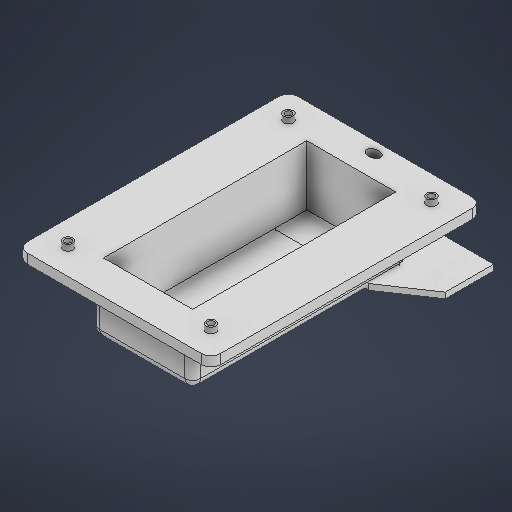
# Autodesk Inventor part: body
Saved by Autodesk Inventor 2027 (Build 310192000, 192)
## iProperties
Created: 2026-05-11
Part Number: body
Material: Generic
Document SubType Name: Modeling
Designer: maksi
Density: 1 g/cm^3
Appearance: Default
Author: maksi
Autodesk Inventor part; units mm, degrees
ref_plane "YZ Plane" through (0, 0, 0) normal (1, 0, 0) x (0, 1, 0)
ref_plane "XZ Plane" through (0, 0, 0) normal (0, 1, 0) x (-1, 0, 0)
ref_plane "XY Plane" through (0, 0, 0) normal (0, 0, 1) x (1, 0, 0)
sketch "Sketch1" plane through (0, 0, 0) normal (0, 1, 0) x (-1, 0, 0)
  line L0 (-40, 60) -> (40, 60)
  line L1 (40, 60) -> (40, -60)
  line L2 (40, -60) -> (-40, -60)
  line L3 (-40, -60) -> (-40, 60)
  line L4 (-40, 60) -> (40, -60) construction
  line L5 (40, 60) -> (-40, -60) construction
  line L6 (40, -60) -> (38.6, -60) construction
  line L7 (38.6, -60) -> (38.6, -58.6) construction
  line L8 (38.6, -58.6) -> (40, -58.6) construction
  line L9 (40, -58.6) -> (40, -60) construction
  line L10 (38.6, -58.6) -> (35.3, -58.6) construction
  line L11 (35.3, -58.6) -> (35.3, -55.3) construction
  line L12 (35.3, -55.3) -> (38.6, -55.3) construction
  line L13 (38.6, -55.3) -> (38.6, -58.6) construction
  circle A0 centre (36.95, -56.95) radius 1.65
  circle A1 centre (-36.95, -56.95) radius 1.65
  circle A2 centre (36.95, 56.95) radius 1.65
  circle A3 centre (-36.95, 56.95) radius 1.65
  line L14 (50, -70) -> (50, 70)
  line L15 (50, 70) -> (-50, 70)
  line L16 (-50, 70) -> (-50, -70)
  line L17 (-50, -70) -> (50, -70)
  line L18 (-23, 52.5) -> (23, 52.5)
  line L19 (23, 52.5) -> (23, -52.5)
  line L20 (23, -52.5) -> (-23, -52.5)
  line L21 (-23, -52.5) -> (-23, 52.5)
  line L22 (-23, 52.5) -> (23, -52.5) construction
  line L23 (23, 52.5) -> (-23, -52.5) construction
  point P0 (0, 0)
  dimension "d0" = 80
  dimension "d1" = 120
  dimension "d2" = 1.4
  dimension "d3" = 1.4
  dimension "d4" = 3.3
  dimension "d5" = 3.3
  dimension "d6" = 3.3
  dimension "d9" = 73.9
  dimension "d12" = 113.9
  dimension "d15" = 10
  dimension "d16" = 46
  dimension "d17" = 105
  constraints: 48 end point, 10 parallel, 5 horizontal, 5 perpendicular, 4 centre point, 4 midpoint, 2 tangent, 1 vertical, 9 other
  measures "d0" distance of L1.end L2.end
  measures "d1" distance of L0.end L1.end
  measures "d2" distance of L7.end L8.end
  measures "d3" distance of L6.end L7.end
  measures "d4" distance of L11.end L12.end
  measures "d5" distance of L10.end L11.end
  measures "d6" diameter of A0
  measures "d9" distance of A0.centre A1.centre
  measures "d12" distance of A0.centre A2.centre
  measures "d15" distance between parallel lines of L1 L14
  measures "d16" distance of L19.end L20.end
  measures "d17" distance of L18.end L19.end
extrude "Extrusion1" add sketch "Sketch1" along normal blind 5 contours L0 L1 L2 L3 | L17 L16 L15 L14
sketch "Sketch2" plane through (-50, 0, 70) normal (0, 0, 1) x (1, 0, 0)
  line L0 (73, 0) -> (27, 0) projected
  line L1 (27, 0) -> (73, 0)
  line L2 (73, 0) -> (73, -26)
  line L3 (73, -26) -> (27, -26)
  line L4 (27, -26) -> (27, 0)
  line L5 (0, 0) -> (100, 0) projected
  line L6 (24, 3) -> (76, 3)
  line L7 (76, 3) -> (76, -25)
  line L8 (72, -29) -> (28, -29)
  line L9 (24, -25) -> (24, 3)
  arc A0 (24, -25) -> (28, -29) centre (28, -25) ccw
  arc A1 (72, -29) -> (76, -25) centre (72, -25) ccw
  point P0 (50, 0)
  point P1 (24, 0)
  point P2 (76, 0)
  dimension "d20" = 26
  dimension "d21" = 3
  dimension "d22" = 4
  constraints: 16 end point, 4 parallel, 4 point on circle, 4 tangent, 2 centre point, 2 perpendicular, 1 collinear, 1 equal radius, 3 other
  measures "d20" distance of L0.start L2.end
  measures "d21" distance between parallel lines of L4 L9
  measures "d22" radius of A0
extrude "Extrusion2" add sketch "Sketch2" against normal up to surface (105 mm away) from surface at -17.5 contours L5 L7 A1 L8 A0 L9 L4 L3 L2
sketch "Sketch3" plane through (23, -26, -52.5) normal (0, 0, -1) x (-1, 0, 0)
  line L0 (-3, 26) -> (-3, 1) projected
  arc A0 (-3, 1) -> (1, -3) centre (1, 1) ccw projected
  line L1 (1, -3) -> (45, -3) projected
  arc A1 (45, -3) -> (49, 1) centre (45, 1) ccw projected
  line L2 (49, 1) -> (49, 26) projected
  line L3 (46, 26) -> (0, 26) projected
  line L4 (-3, 26) -> (0, 26) projected
  line L5 (46, 26) -> (49, 26) projected
  point P0 (23, 26)
extrude "Extrusion3" add sketch "Sketch3" along normal blind 3
extrude "Extrusion4" add sketch "Sketch3" against normal blind 3 from surface at -105
fillet "Fillet1" radius 4 10 edges at (26, -12.5, 55.5) (0, -29, 55.5) (-24.8284, -27.8284, 55.5) (-26, -12.5, 55.5) (24.8284, -27.8284, 55.5) (0, -29, -55.5) (-24.8284, -27.8284, -55.5) (-26, -12.5, -55.5) (26, -12.5, -55.5) (24.8284, -27.8284, -55.5)
sketch "Sketch4" plane through (0, 5, 0) normal (0, 1, 0) x (1, 0, 0)
  circle A0 centre (-36.95, 56.95) radius 1.65 projected
  circle A1 centre (-36.95, 56.95) radius 2.5
  circle A2 centre (-36.95, 56.95) radius 1.65
  point P0 (0, 0)
  dimension "d30" = 5
  constraints: 2 centre point, 2 coincident
  measures "d30" diameter of A1
extrude "Extrusion5" add sketch "Sketch4" along normal blind 3
pattern_linear "Rectangular Pattern1" count 2 spacing 73.9 along (1, 0, 0) count 2 spacing 113.9 along (0, 0, 1) of "Extrusion5"
fillet "Fillet2" radius 5 4 edges at (-50, 2.5, 70) (-50, 2.5, -70) (50, 2.5, -70) (50, 2.5, 70)
sketch "Sketch5" plane through (-22, -29, -51.5) normal (0, -1, 0) x (1, 0, 0)
  line L0 (44, 0) -> (44, -4) projected
  line L1 (44, 0) -> (71.6, 0)
  line L2 (71.6, 0) -> (71.6, -25)
  line L3 (71.6, -25) -> (44, -25)
  line L4 (44, -25) -> (44, 0)
  line L5 (44, 0) -> (0, 0) projected
  line L6 (0, 0) -> (-27.6, 0)
  line L7 (-27.6, 0) -> (-27.6, -25)
  line L8 (-27.6, -25) -> (0, -25)
  line L9 (0, -25) -> (0, 0)
  line L10 (44, -25) -> (0, -25)
  line L11 (0, -25) -> (0, 0)
  line L12 (0, 0) -> (44, 0)
  line L13 (44, 0) -> (44, -25)
  line L14 (44, -25) -> (0, 0) construction
  line L15 (0, -25) -> (44, 0) construction
  ellipse E0 centre (22, -12.5) end of major axis (18.3001, -12.5) minor radius 2.5167
  line L16 (-1, -1) -> (45, -1) projected
  line L17 (0, 0) -> (-4, 0) projected
  line L18 (0, 103) -> (0, 0) projected
  line L19 (-4, 103) -> (0, 103) projected
  line L20 (-4, 103) -> (-4, 0) projected
  line L21 (48, 0) -> (44, 0) projected
  line L22 (48, 103) -> (48, 0) projected
  line L23 (44, 103) -> (48, 103) projected
  line L24 (44, 103) -> (44, 0) projected
  line L25 (-27.6, 0) -> (0, 15.9349)
  line L26 (-27.6, 0) -> (4.2697, 0) construction
  line L27 (0, 15.9349) -> (48, 15.9349)
  line L28 (48, 103) -> (48, 0) projected
  line L29 (48, 15.9349) -> (71.6, 0)
  point P0 (22, 51.5)
  dimension "d40" = 27.6
  dimension "d41" = 25
  dimension "d42" = 27.6
  dimension "d43" = 25
  dimension "d44" = 30
  constraints: 36 end point, 6 parallel, 5 horizontal, 4 perpendicular, 2 point on line, 1 equal length, 1 midpoint, 2 other
  measures "d40" distance of L2.end L3.end
  measures "d41" distance of L1.end L2.end
  measures "d42" distance of L8.end L7.end
  measures "d43" distance of L7.end L6.end
  measures "d44" angle of L26 L25
extrude "Extrusion6" add sketch "Sketch5" against normal blind 3 separate body contours L1 L2 L3 L4 L0 | L24 L27 L22 L1 | L0 L16 L9 L5 | L5 L18 L27 L24 | L0 L4 L10 L9 L16 | L22 L29 L1 | L9 L8 L7 L6 | L6 L20 L25 L18 | L6 L25 L20
sketch "Sketch6" plane through (0, 5, 0) normal (0, 1, 0) x (1, 0, 0)
  ellipse E0 centre (0, 64) end of major axis (3.6999, 64) minor radius 2.5167 projected
  point P0 (0, 0)
extrude "Extrusion7" cut sketch "Sketch6" against normal through all bodies 1
body "Solid1"
body "Solid2"
